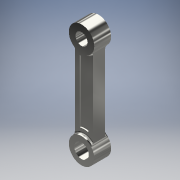
# Autodesk Inventor part: Component 6 (Connecting Rod)
Saved by Autodesk Inventor 2018 (Build 220112000, 112)
## iProperties
Created: 2023-03-14
Part Number: Component 6 (Connecting Rod)
Material: Generic
Document SubType Name: Modeling
Designer: Habib Mohamed
Density: 1 g/cm^3
Appearance: Silicon Nitride - Polished
Author: Habib Mohamed
Autodesk Inventor part; units mm, degrees
ref_plane "YZ Plane" through (0, 0, 0) normal (1, 0, 0) x (0, 1, 0)
ref_plane "XZ Plane" through (0, 0, 0) normal (0, 1, 0) x (-1, 0, 0)
ref_plane "XY Plane" through (0, 0, 0) normal (0, 0, 1) x (1, 0, 0)
sketch "Sketch1" plane through (0, 0, 0) normal (0, 0, 1) x (1, 0, 0)
  line L0 (0, 0) -> (0, 40) construction
  circle A0 centre (0, 40) radius 2.5
  circle A1 centre (0, 40) radius 5.25
  circle A2 centre (0, 0) radius 3
  circle A3 centre (0, 0) radius 5.25
  dimension "d0" = 40
  dimension "d1" = 5
  dimension "d2" = 10.5
  dimension "d3" = 6
  dimension "d4" = 10.5
  constraints: 4 centre point, 4 coincident, 2 end point, 1 vertical
  measures "d0" distance of L0.start L0.end
  measures "d1" diameter of A0
  measures "d2" diameter of A1
  measures "d3" diameter of A2
  measures "d4" diameter of A3
extrude "Extrusion1" add sketch "Sketch1" along normal mid plane 7
sketch "Sketch2" plane through (0, 0, 0) normal (0, 0, 1) x (1, 0, 0)
  circle A0 centre (0, 40) radius 2.5 projected
  circle A1 centre (0, 40) radius 5.25 projected
  circle A2 centre (0, 0) radius 3 projected
  circle A3 centre (0, 0) radius 5.25 projected
  circle A4 centre (0, 0) radius 3 projected
  line L0 (0, 40) -> (0, 0) construction
  line L1 (-3.75, 36.3258) -> (-3.75, 3.6742)
  line L2 (3.75, 36.3258) -> (3.75, 3.6742)
  point P0 (-3.75, 40)
  point P1 (-3.75, 0)
  point P2 (3.75, 40)
  point P3 (3.75, 0)
  dimension "d7" = 3.75
  constraints: 6 end point, 4 point on circle, 3 parallel, 2 symmetric about line, 1 vertical
  measures "d7" distance between parallel lines of L0 L1
extrude "Extrusion2" add sketch "Sketch2" along normal mid plane 5 contours A1 L2 A3 L1
sketch "Sketch3" plane through (0, 0, 2.5) normal (0, 0, 1) x (1, 0, 0)
  line L0 (-3.75, 36.3258) -> (-3.75, 3.6742) projected
  line L1 (-3.75, 36.3258) -> (-3.75, 3.6742) projected
  arc A0 (3.75, 3.6742) -> (-3.75, 3.6742) centre (0, 0) ccw projected
  line L2 (3.75, 3.6742) -> (3.75, 36.3258) projected
  arc A1 (-3.75, 36.3258) -> (3.75, 36.3258) centre (0, 40) ccw projected
  line L3 (1.75, 32.9644) -> (1.75, 7.0356)
  arc A2 (1.75, 7.0356) -> (-1.75, 7.0356) centre (0, 0) ccw
  line L4 (-1.75, 7.0356) -> (-1.75, 32.9644)
  arc A3 (-1.75, 32.9644) -> (1.75, 32.9644) centre (0, 40) ccw
  dimension "d10" = 2
  constraints: 4 end point, 4 point on circle, 2 centre point, 3 other
  measures "d10" distance between parallel lines of L2 L3
extrude "Extrusion3" cut sketch "Sketch3" against normal blind 0.5 contours L3 A2 L4 A3
mirror "Mirror1" about plane through (0, 0, 0) normal (0, 0, 1) of "Extrusion3"
fillet "Fillet1" radius 0.75 8 edges at (0, 34.75, 2.5) (3.75, 36.3258, 0) (0, 34.75, -2.5) (-3.75, 36.3258, 0) (3.75, 3.6742, 0) (0, 5.25, -2.5) (-3.75, 3.6742, 0) (0, 5.25, 2.5)
body "Solid1"
